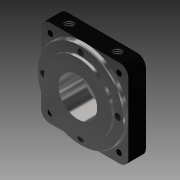
# Autodesk Inventor part: P80 Front Block
Saved by Autodesk Inventor 2013 (Build 170138000, 138)
## iProperties
Created: 2013-02-10
Part Number: P80 Front Block
Material: Steel
Document SubType Name: Modeling
Designer: Moses
Density: 7.85 g/cm^3
Mass: 387.783 g
Surface Area: 147.32 cm^2
Volume: 49.3991 cm^3
Author: Moses
Autodesk Inventor part; units mm, degrees
ref_plane "YZ Plane" through (0, 0, 0) normal (1, 0, 0) x (0, 1, 0)
ref_plane "XZ Plane" through (0, 0, 0) normal (0, 1, 0) x (-1, 0, 0)
ref_plane "XY Plane" through (0, 0, 0) normal (0, 0, 1) x (1, 0, 0)
sketch "Sketch1" plane through (0, 0, 0) normal (0, 0, 1) x (1, 0, 0)
  circle A0 centre (0, 0) radius 14
  line L0 (-31.75, 31.75) -> (31.75, 31.75)
  line L1 (31.75, 31.75) -> (31.75, -31.75)
  line L2 (31.75, -31.75) -> (-31.75, -31.75)
  line L3 (-31.75, -31.75) -> (-31.75, 31.75)
  circle A1 centre (0, 27.0002) radius 2.3495
  line L4 (-31.75, 0) -> (31.75, 0) construction
  line L5 (0, 31.75) -> (0, -31.75) construction
  circle A2 centre (-27.0002, 0) radius 2.3495
  circle A3 centre (27.0002, 0) radius 2.3495
  circle A4 centre (0, -27.0002) radius 2.3495
  circle A5 centre (-25.0002, 25.0002) radius 2
  line L6 (-27.0002, -27.0002) -> (27.0002, -27.0002) construction
  line L7 (27.0002, -27.0002) -> (27.0002, 27.0002) construction
  line L8 (27.0002, 27.0002) -> (-27.0002, 27.0002) construction
  line L9 (-27.0002, 27.0002) -> (-27.0002, -27.0002) construction
  circle A6 centre (-25.0002, 25.0002) radius 3.5
  circle A7 centre (25.0002, 25.0002) radius 2
  circle A8 centre (25.0002, 25.0002) radius 3.5
  circle A9 centre (-25.0002, -25.0002) radius 2
  circle A10 centre (-25.0002, -25.0002) radius 3.5
  circle A11 centre (25.0002, -25.0002) radius 2
  circle A12 centre (25.0002, -25.0002) radius 3.5
  dimension "d2" = 28
  dimension "d7" = 63.5
  dimension "d8" = 63.5
  dimension "d9" = 27.0002
  dimension "d10" = 4.699
  dimension "d11" = 27.0002
  dimension "d12" = 27.0002
  dimension "d13" = 27.0002
  dimension "d14" = 54.0004
  dimension "d17" = 4
  dimension "d18" = 7
  constraints: 20 end point, 13 centre point, 9 equal radius, 8 tangent, 7 midpoint, 6 coincident, 4 parallel, 4 point on line, 2 horizontal, 2 perpendicular
  measures "d2" diameter of A0
  measures "d7" distance of L0.end L1.end
  measures "d8" distance of L1.end L2.end
  measures "d9" distance of A1.centre point (0, 0)
  measures "d10" diameter of A1
  measures "d11" distance of point (0, 0) A2.centre
  measures "d12" distance of A3.centre point (0, 0)
  measures "d13" distance of A4.centre point (0, 0)
  measures "d14" distance of A3.centre A2.centre
  measures "d17" diameter of A5
  measures "d18" diameter of A6
extrude "Extrusion1" add sketch "Sketch1" along normal blind 12.7 contours L0 L1 L2 L3 | A6 | A8 | A10 | A12
extrude "Extrusion2" cut sketch "Sketch1" along normal blind 4 contours A6 | A8 | A10 | A12
fillet "Fillet1" radius 6.35 4 edges at (31.75, 31.75, 6.35) (-31.75, 31.75, 6.35) (31.75, -31.75, 6.35) (-31.75, -31.75, 6.35)
sketch "Sketch2" plane through (0, 0, 12.7) normal (0, 0, 1) x (1, 0, 0)
  circle A0 centre (0, 0) radius 14 projected
  circle A1 centre (0, -27.0002) radius 2.3495 projected
  circle A2 centre (27.0002, 0) radius 2.3495 projected
  circle A3 centre (-27.0002, 0) radius 2.3495 projected
  circle A4 centre (0, 27.0002) radius 2.3495 projected
  circle A5 centre (0, 0) radius 31.75
  dimension "d22" = 63.5
  constraints: 1 centre point, 1 coincident
  measures "d22" diameter of A5
extrude "Extrusion3" add sketch "Sketch2" along normal blind 3
sketch "Sketch3" plane through (0, 0, 15.7) normal (0, 0, 1) x (1, 0, 0)
  circle A0 centre (0, 0) radius 14 projected
  circle A1 centre (27.0002, 0) radius 2.3495 projected
  circle A2 centre (0, 0) radius 31.75 projected
  circle A3 centre (0, 0) radius 24.6507
  constraints: 1 centre point, 1 coincident, 1 tangent
extrude "Extrusion4" add sketch "Sketch3" along normal blind 2 contours A3
thread "Thread1" size "10-32 UNF" class "2B" standard "ANSI Unified Screw Threads" full length
thread "Thread2" size "10-32 UNF" class "2B" standard "ANSI Unified Screw Threads" full length
thread "Thread3" size "10-32 UNF" class "2B" standard "ANSI Unified Screw Threads" full length
thread "Thread4" size "10-32 UNF" class "2B" standard "ANSI Unified Screw Threads" full length
chamfer "Chamfer1" distance 0.635 angle 45 1 edges at (-31.75, 0, 15.7)
sketch "Sketch4" plane through (-25.4, 31.75, 0) normal (0, 1, 0) x (1, 0, 0)
  line L0 (50.8, -12.7) -> (25.4, -12.7) projected
  line L1 (25.4, 0) -> (25.4, -12.7) construction
  line L2 (7.8994, -6.35) -> (42.9006, -6.35) construction
  circle A0 centre (7.8994, -6.35) radius 3.175
  circle A1 centre (42.9006, -6.35) radius 3.175
  point P0 (25.4, -6.35)
  dimension "d38" = 35.0012
  dimension "d40" = 6.35
  constraints: 4 end point, 2 centre point, 2 coincident, 2 midpoint, 2 perpendicular, 1 equal radius
  measures "d38" distance of L2.start L2.end
  measures "d40" diameter of A0
extrude "Extrusion5" cut sketch "Sketch4" against normal blind 12.7
sketch "Sketch5" plane through (-25.4, -31.75, 0) normal (0, -1, 0) x (1, 0, 0)
  line L0 (0, 12.7) -> (25.4, 12.7) projected
  line L1 (25.4, 0) -> (25.4, 12.7) construction
  line L2 (7.8994, 6.35) -> (42.9006, 6.35) construction
  circle A0 centre (7.8994, 6.35) radius 3.175
  circle A1 centre (42.9006, 6.35) radius 3.175
  point P0 (25.4, 6.35)
  dimension "d43" = 35.0012
  dimension "d45" = 6.35
  constraints: 4 end point, 2 centre point, 2 coincident, 2 midpoint, 2 perpendicular, 1 equal radius
  measures "d43" distance of L2.start L2.end
  measures "d45" diameter of A0
extrude "Extrusion6" cut sketch "Sketch5" against normal blind 12.7
thread "Thread5" size "1/4-20 UNC" class "2B" standard "ANSI Unified Screw Threads" full length
thread "Thread6" size "1/4-20 UNC" class "2B" standard "ANSI Unified Screw Threads" full length
thread "Thread7" size "1/4-20 UNC" class "2B" standard "ANSI Unified Screw Threads" full length
thread "Thread8" size "1/4-20 UNC" class "2B" standard "ANSI Unified Screw Threads" full length
equation "\"d11\" = d9"
equation "\"d12\" = d9"
equation "\"d13\" = d9"
body "Solid1"
